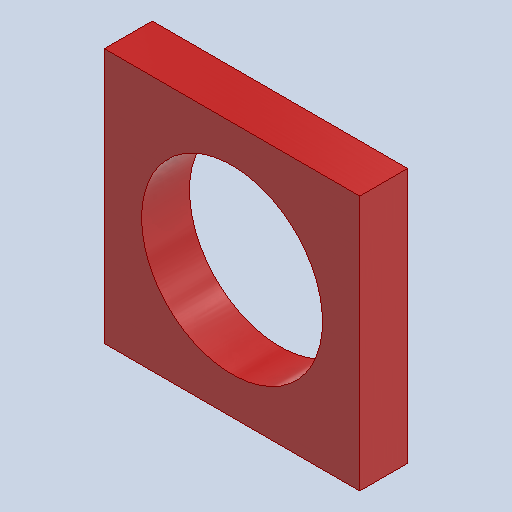
# Autodesk Inventor part: Bobina
Saved by Autodesk Inventor 2022 (Build 260153000, 153)
## iProperties
Created: 2022-03-23
Part Number: Bobina
Material: Genérico
Document SubType Name: Modeling
Designer: aarco
Density: 1 g/cm^3
Appearance: Rojo
Mass: 58135.1 g
Surface Area: 15222.9 cm^2
Volume: 58135.1 cm^3
Author: aarco
Autodesk Inventor part; units mm, degrees
ref_plane "YZ Plane" through (0, 0, 0) normal (1, 0, 0) x (0, 1, 0)
ref_plane "XZ Plane" through (0, 0, 0) normal (0, 1, 0) x (-1, 0, 0)
ref_plane "XY Plane" through (0, 0, 0) normal (0, 0, 1) x (1, 0, 0)
sketch "Boceto1" plane through (0, 0, 0) normal (0, 0, 1) x (1, 0, 0)
  line L0 (-400, 800) -> (400, 800)
  line L1 (400, 800) -> (400, 0)
  line L2 (400, 0) -> (-400, 0)
  line L3 (-400, 0) -> (-400, 800)
  circle A0 centre (0, 400) radius 283.4638
  line L4 (-400, 400) -> (400, 400)
  point P0 (0, 0)
  point P1 (0, 0)
  dimension "d0" = 800
  constraints: 10 end point, 4 midpoint, 2 coincident, 2 parallel, 2 perpendicular, 1 centre point, 1 horizontal
  measures "d0" distance of L0.start L0.end
extrude "Extrusión1" add sketch "Boceto1" along normal blind 150 contours L0 L1 L4 A0 L3 | L4 A0 L1 L2 L3
